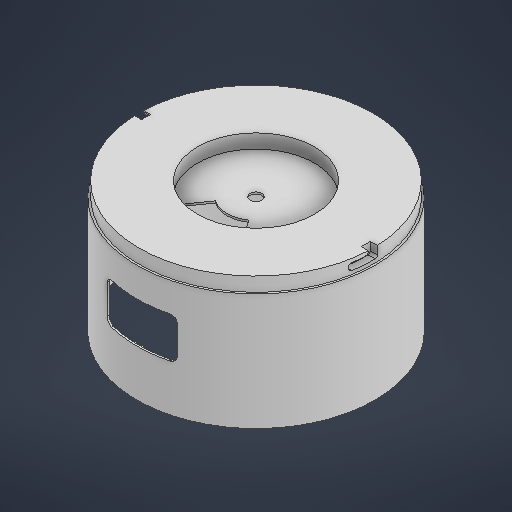
# Autodesk Inventor part: base
Saved by Autodesk Inventor 2025.1 (Build 291241020, 241B)
## iProperties
Created: 2024-09-16
Part Number: base
Material: Generic
Document SubType Name: Modeling
Designer: maxim
Density: 1 g/cm^3
Appearance: Default
Author: maxim
Autodesk Inventor part; units mm, degrees
sketch "base" plane through (0, 0, 0) normal (0, 0, 1) x (1, 0, 0)
  line L0 (0, 0) -> (-102, 0)
  line L1 (-102, 0) -> (-102, 100)
  line L2 (-50.1, 112) -> (-50.1, 100)
  line L3 (-50.1, 100) -> (0, 100)
  line L4 (0, 0) -> (0, 181.0231)
  line L5 (-50.1, 100) -> (-102, 100)
  line L6 (-50.1, 112) -> (-100.275, 112)
  line L7 (-100.275, 112) -> (-100.275, 100)
  point P0 (-50.1, 106)
  dimension "BaseRadius" = 102
  dimension "BaseHeight" = 100
  dimension "BaseRotorMargin" = 12
  dimension "BaseFeedRadius" = 100.2
  dimension "d57" = 1.725
  dimension "d58" = 200.55
  constraints: 16 end point, 5 perpendicular, 2 horizontal, 2 point on line, 1 midpoint, 1 vertical
  measures "BaseRadius" distance of L0.start L0.end
  measures "BaseHeight" distance of L0.end L1.end
  measures "BaseRotorMargin" distance of L2.start L2.end
  measures "BaseFeedRadius" diameter of point (-50.1, 106) L4
  measures "d57" distance from line of L1.end L7
  measures "d58" diameter of L7 L4
revolve "Revolution1" add sketch "base" angle 360 about axis through (0, 0, 0) along (0, 1, 0) contours L0 L1 L5 L3 L4
shell "Shell2" thickness 1.6 removed faces 1 at (-23.2432, 0, 54.3964)
revolve "Revolution2" add sketch "base" angle 360 about axis through (0, 0, 0) along (0, 1, 0) contours L5 L7 L6 L2
sketch "Sketch4" plane through (0, 100, 0) normal (0, 1, 0) x (1, 0, 0)
  point P0 (0, 0)
  point P1 (0, 0)
  constraints: 1 coincident
hole "Hole2" at (0, 100, 0) direction (0, -1, 0) diameter 10.2 end through all
ref_plane "Work Plane1" through (0, 0, 150) normal (0, 0, 1) x (1, 0, 0)
sketch "Sketch5" plane through (0, 0, 150) normal (0, 0, 1) x (1, 0, 0)
  line L0 (-25, 75) -> (25, 75)
  line L1 (30, 70) -> (30, 45)
  line L2 (25, 40) -> (-25, 40)
  line L3 (-30, 45) -> (-30, 70)
  arc A0 (-25, 75) -> (-30, 70) centre (-25, 70) ccw
  arc A1 (-30, 45) -> (-25, 40) centre (-25, 45) ccw
  arc A2 (30, 70) -> (25, 75) centre (25, 70) ccw
  arc A3 (25, 40) -> (30, 45) centre (25, 45) ccw
  line L4 (0, 0) -> (0, 181.0231) projected
  line L5 (102, 0) -> (-102, 0) projected
  point P0 (0, 75)
  point P1 (102, 100)
  point P2 (-102, 100)
  dimension "d26" = 5
  dimension "d27" = 50
  dimension "d28" = 25
  constraints: 8 end point, 8 point on circle, 8 tangent, 4 centre point, 3 equal radius, 2 parallel, 1 horizontal, 1 midpoint, 1 perpendicular, 1 point on line
  measures "d26" radius of A0
  measures "d27" distance of L0.start L0.end
  measures "d28" distance of L1.start L1.end
extrude "Extrusion2" cut sketch "Sketch5" against normal up to next
sketch "Sketch6" plane through (0, 98.4, 0) normal (0, -1, 0) x (1, 0, 0)
  arc A0 (0, 50.1) -> (-28.7362, 41.0395) centre (0, 0) ccw
  line L0 (0, 0) -> (-28.7362, 41.0395)
  line L1 (0, 0) -> (0, 133.4499)
  arc A1 (28.7362, 41.0395) -> (0, 50.1) centre (0, 0) ccw
  line L2 (0, 0) -> (28.7362, 41.0395)
  line L3 (0, 22.9733) -> (-16.0861, 22.9733) construction
  line L4 (0, 22.9733) -> (16.0861, 22.9733) construction
  arc A2 (14.3394, 20.4788) -> (-14.3394, 20.4788) centre (0, 0) ccw
  point P0 (0, 0)
  point P1 (0, 25.05)
  point P2 (0, 25)
  dimension "d34" = 50.1
  dimension "d98" = 70
  dimension "d99" = 25
  constraints: 10 end point, 8 point on line, 7 point on circle, 3 centre point, 2 coincident, 1 collinear, 1 perpendicular, 1 vertical
  measures "d34" distance of L0.start L0.end
  measures "d98" angle of L2 L0
  measures "d99" distance of L1.start point (0, 25)
extrude "Extrusion3" cut sketch "Sketch6" against normal up to next contours L1 A2 L0 A0 | A1 L2 A2 L1
sketch "LoftSketch" plane through (0, 98.4, 0) normal (0, -1, 0) x (1, 0, 0)
  line L0 (0, 10) -> (-25, 10)
  line L1 (-30, 15) -> (-30, 50)
  line L2 (-25, 55) -> (0, 55)
  line L3 (0, 0) -> (0, 133.4499) projected
  line L4 (0, 10) -> (25, 10)
  line L5 (30, 15) -> (30, 50)
  line L6 (25, 55) -> (0, 55)
  arc A0 (-30, 15) -> (-25, 10) centre (-25, 15) ccw
  arc A1 (-25, 55) -> (-30, 50) centre (-25, 50) ccw
  arc A2 (25, 10) -> (30, 15) centre (25, 15) ccw
  arc A3 (30, 50) -> (25, 55) centre (25, 50) ccw
  point P0 (0, 0)
  point P1 (-30, 55)
  point P2 (-30, 10)
  point P3 (30, 55)
  point P4 (30, 10)
  dimension "d38" = 10
  dimension "d39" = 30
  dimension "d40" = 45
  dimension "d49" = 5
  dimension "d50" = 5
  constraints: 12 end point, 8 point on circle, 8 point on line, 8 tangent, 4 centre point, 2 equal radius, 2 symmetric about line, 1 horizontal, 1 parallel, 1 perpendicular
  measures "d38" distance of point (0, 0) L0.start
  measures "d39" distance of point (-30, 55) L2.end
  measures "d40" distance of point (-30, 10) point (-30, 55)
  measures "d49" radius of A0
  measures "d50" radius of A2
surface_loft "LoftSrf2"
ref_plane "Work Plane4" through (25, 38, 97.2376) normal (0, 1, 0) x (1, 0, 0)
ref_plane "Work Plane3" through (25, 40, 97.2376) normal (0, 1, 0) x (1, 0, 0)
sketch "Sketch10" plane through (25, 38, 97.2376) normal (0, 1, 0) x (1, 0, 0)
  circle A0 centre (-25, 97.2376) radius 102 projected
  line L0 (-35.5899, -4.2111) -> (-14.4101, -4.2111)
  line L1 (-14.4101, -4.2111) -> (-14.4101, -0.2111)
  line L2 (-14.4101, -0.2111) -> (-35.5899, -0.2111)
  line L3 (-35.5899, -0.2111) -> (-35.5899, -4.2111)
  dimension "d61" = 4
  constraints: 8 end point, 2 parallel, 2 point on circle, 1 horizontal, 1 perpendicular
  measures "d61" distance of L0.end L1.end
extrude "Extrusion4" add sketch "Sketch10" against normal blind 4 contours L3 L2 L1 L0
sketch "Sketch11" plane through (10.5899, 38, 99.8399) normal (1, 0, 0) x (0, 0, -1)
  line L0 (0, -4) -> (0, -4) projected
  line L1 (0, -4) -> (2.3912, -4) projected
  line L2 (2.3912, -4) -> (0, -4) projected
  line L3 (2.3912, 0) -> (2.3912, -4) projected
  line L4 (2.3912, 0) -> (2.3912, -4) projected
  line L5 (2.3912, 0) -> (0, -4)
  point P0 (99.8399, -38)
  constraints: 2 end point
extrude "Extrusion5" cut sketch "Sketch11" against normal up to surface (21.1797 mm away)
ref_plane "Work Plane5" through (0, 106, 0) normal (0, 1, 0) x (1, 0, 0)
sketch "Sketch13" plane through (0, 106, 0) normal (0, 1, 0) x (1, 0, 0)
  circle A0 centre (0, 0) radius 100.275 projected
  circle A1 centre (0, 0) radius 100.275 projected
  line L0 (0, 0) -> (-100.1952, -4)
  line L1 (0, 0) -> (-100.1952, 4)
  line L2 (0, 0) -> (-100.275, 0) construction
  line L3 (-86.9841, 0) -> (-86.9841, 3.4726) construction
  line L4 (-86.9841, 0) -> (-86.9841, -3.4726) construction
  line L5 (0, 0) -> (-98.4585, 19)
  circle A2 centre (0, 0) radius 5.1 projected
  circle A3 centre (0, 0) radius 94.275
  point P0 (-100.1952, -4)
  point P1 (-100.1952, 4)
  point P2 (-94.2, -3.7607)
  point P3 (-92.5672, 17.8631)
  point P4 (-94.2, 3.7607)
  point P5 (2.9252, -4.1777)
  point P6 (-2.9252, -4.1777)
  dimension "d76" = 8
  dimension "d77" = 15
  dimension "d90" = 6
  constraints: 12 end point, 4 point on circle, 4 point on line, 1 centre point, 1 coincident, 1 collinear, 1 horizontal, 1 perpendicular
  measures "d76" distance of L0.end L1.end
  measures "d77" vertical distance of L1.end L5.end
  measures "d90" radial gap between concentric circles of A0 A3
extrude "Extrusion6" cut sketch "Sketch13" along normal mid plane 6 contours L5 A3 L1 A0 | A0 L1 A3 L0
extrude "Extrusion8" cut sketch "Sketch13" along normal through all contours A0 L1 A3 L0
fillet "Fillet4" radius 2 1 edges at (-97.1976, 109, -3.8803)
fillet "Fillet5" radius 2 3 edges at (-95.5128, 109, -18.4316) (-95.5128, 103, -18.4316) (-97.1976, 103, 3.8803)
pattern_circular "Circular Pattern2" count 2 over 360 about axis through (0, 106, 0) along (0, 1, 0) of "Extrusion6", "Extrusion8", "Fillet4", "Fillet5"
body "Solid2"
body "Srf2"
